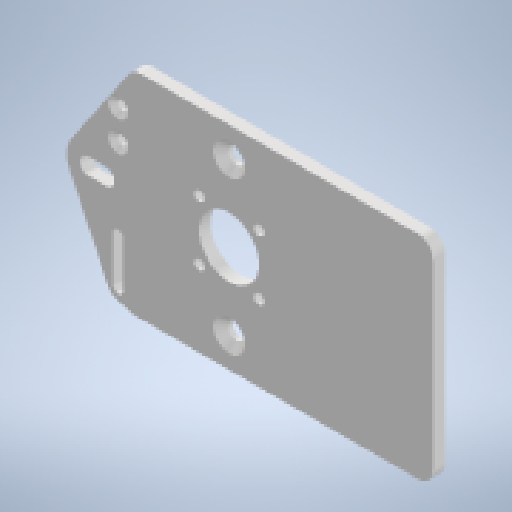
# Autodesk Inventor part: plate_3
Saved by Autodesk Inventor 2024 (Build 280153000, 153)
## iProperties
Created: 2026-02-08
Part Number: plate_3
Material: Generic
Document SubType Name: Modeling
Designer: SEMEN
Density: 1 g/cm^3
Appearance: Default
Author: SEMEN
Autodesk Inventor part; units mm, degrees
ref_plane "YZ Plane" through (0, 0, 0) normal (1, 0, 0) x (0, 1, 0)
ref_plane "XZ Plane" through (0, 0, 0) normal (0, 1, 0) x (-1, 0, 0)
ref_plane "XY Plane" through (0, 0, 0) normal (0, 0, 1) x (1, 0, 0)
sketch "Sketch1" plane through (0, 0, 0) normal (0, 0, 1) x (1, 0, 0)
  circle A0 centre (13.407, 27.6606) radius 2.5 construction
  circle A1 centre (13.407, 27.6606) radius 10 projected
  circle A2 centre (57.407, 53.064) radius 2.5 construction
  circle A3 centre (57.407, 53.064) radius 10 construction
  circle A4 centre (57.407, 2.2572) radius 2.5 construction
  circle A5 centre (57.407, 2.2572) radius 10 construction
  line L0 (125.407, 63.064) -> (125.407, -7.7428)
  line L1 (125.407, -7.7428) -> (25.407, -7.7428)
  line L2 (125.407, 82.5038) -> (125.407, 159.5038) projected
  line L3 (57.407, 53.064) -> (57.407, 2.2572) construction
  circle A6 centre (57.407, 27.6606) radius 10
  line L4 (47.1446, 17.3983) -> (70.9177, 41.1714) construction
  circle A7 centre (47.5075, 17.7611) radius 4 construction
  circle A8 centre (67.3065, 37.5601) radius 4 construction
  line L5 (45.5703, 39.4972) -> (72.2419, 12.8257) construction
  circle A9 centre (47.5075, 37.5601) radius 4 construction
  circle A10 centre (67.3065, 17.7611) radius 4 construction
  line L6 (25.407, -109.9962) -> (25.407, 140.0038) projected
  line L7 (25.407, 63.064) -> (125.407, 63.064)
  line L8 (20.907, -0.3966) -> (20.907, 57.2182) construction
  line L9 (20.907, -1.9538) -> (20.907, 13.0462) construction
  line L10 (22.707, -1.9538) -> (22.707, 13.0462)
  line L11 (19.107, 13.0462) -> (19.107, -1.9538)
  arc A11 (19.107, -1.9538) -> (22.707, -1.9538) centre (20.907, -1.9538) ccw
  arc A12 (22.707, 13.0462) -> (19.107, 13.0462) centre (20.907, 13.0462) ccw
  circle A13 centre (20.907, -1.9538) radius 3.5
  line L12 (25.407, -7.7428) -> (19.5041, -5.1603)
  line L13 (17.7746, -3.5153) -> (4.4573, 23.1992)
  circle A14 centre (20.907, 50.6606) radius 4
  line L14 (25.407, 63.064) -> (17.7373, 53.1005)
  line L15 (4.9656, 33.0219) -> (17.5304, 52.8051)
  point P0 (0, 0)
  point P1 (57.407, 63.064)
  point P2 (57.407, -7.7428)
  point P3 (20.907, 40.6606)
  point P4 (20.907, 5.5462)
  point P5 (20.907, 21.0462)
  dimension "d1" = 20
  dimension "d2" = 45
  dimension "d3" = 8
  dimension "d4" = 8
  dimension "d5" = 45
  dimension "d6" = 8
  dimension "d7" = 8
  dimension "d29" = 4.5
  dimension "d30" = 10
  dimension "d31" = 15
  dimension "d32" = 3.6
  dimension "d33" = 8
  dimension "d34" = 7
  dimension "d43" = 13
  dimension "d44" = 8
  constraints: 30 end point, 16 tangent, 14 point on line, 11 point on circle, 9 centre point, 6 coincident, 2 midpoint, 2 parallel, 2 vertical, 1 collinear, 1 horizontal, 1 perpendicular
  measures "d1" diameter of A6
  measures "d2" angle of L3 L4
  measures "d3" diameter of A7
  measures "d4" diameter of A8
  measures "d5" angle of L3 L5
  measures "d6" diameter of A9
  measures "d7" diameter of A10
  measures "d29" distance between parallel lines of L6 L8
  measures "d30" distance of point (20.907, 50.661) point (20.907, 40.661)
  measures "d31" distance of L9.start L9.end
  measures "d32" diameter of A12
  measures "d33" distance of A1.start L9.end
  measures "d34" diameter of A13
  measures "d43" vertical distance of A1.centre point (20.907, 40.661)
  measures "d44" diameter of A14
extrude "Extrusion1" add sketch "Sketch1" along normal blind 4 contours A1 | A1 L15 A14 L14 L6 L12 A13 L10 A12 L11 L13 | A14 | A13 L11 A11 L10 | L7 L0 L1 L6 picked at (18.8791, -0.1313)
fillet "Fillet1" radius 5 4 edges at (25.407, -7.7428, 2) (25.407, 63.064, 2) (125.407, 63.064, 2) (125.407, -7.7428, 2)
hole "Hole1" at (67.3065, 37.5601, 0) at (47.5075, 37.5601, 0) at (47.5075, 17.7611, 0) at (67.3065, 17.7611, 0) direction (0, 0, 1) diameter 3.4 end through all countersink diameter 6.6 countersink angle 90 clearance for "Countersunk Head GOST 12876-67" size "M3" standard "GOST"
sketch "Sketch2" plane through (0, 0, 4) normal (0, 0, 1) x (1, 0, 0)
  circle A0 centre (13.407, 27.6606) radius 2.5 projected
  circle A1 centre (57.407, 2.2572) radius 2.5 projected
  circle A2 centre (57.407, 53.064) radius 2.5 projected
  line L0 (10.407, 27.6606) -> (16.407, 27.6606) construction
  line L1 (10.407, 24.9106) -> (16.407, 24.9106)
  line L2 (16.407, 30.4106) -> (10.407, 30.4106)
  arc A3 (10.407, 30.4106) -> (10.407, 24.9106) centre (10.407, 27.6606) ccw
  arc A4 (16.407, 24.9106) -> (16.407, 30.4106) centre (16.407, 27.6606) ccw
  point P0 (0, 0)
  dimension "d25" = 3
  dimension "d26" = 5.5
  constraints: 8 end point, 4 point on circle, 4 tangent, 2 centre point, 1 horizontal, 1 midpoint, 1 parallel
  measures "d25" distance of A0.centre L0.end
  measures "d26" diameter of A4
hole "Hole2" at (57.407, 53.064, 4) at (57.407, 2.2572, 4) direction (0, 0, -1) diameter 5.5 end through all countersink diameter 10.4 countersink angle 90 clearance for "Countersunk Head GOST 12876-67" size "M5" standard "GOST"
sketch "Sketch3" plane through (0, 0, 4) normal (0, 0, 1) x (1, 0, 0)
  arc A0 (10.407, 30.4106) -> (10.407, 24.9106) centre (10.407, 27.6606) ccw projected
  line L0 (16.407, 30.4106) -> (10.407, 30.4106) projected
  line L1 (10.407, 24.9106) -> (16.407, 24.9106) projected
  arc A1 (16.407, 24.9106) -> (16.407, 30.4106) centre (16.407, 27.6606) ccw projected
  point P0 (0, 0)
extrude "Extrusion2" cut sketch "Sketch3" against normal up to surface (4 mm away)
sketch "Sketch4" plane through (0, 0, 4) normal (0, 0, 1) x (1, 0, 0)
  point P0 (0, 0)
  point P1 (20.907, 40.6606)
  point P2 (20.907, 50.6606)
hole "Hole3" at (20.907, 40.6606, 4) at (20.907, 50.6606, 4) direction (0, 0, -1) diameter 3.4 end through all countersink diameter 6.6 countersink angle 90 clearance for "Countersunk Head GOST 12876-67" size "M3" standard "GOST"
body "Solid1"
